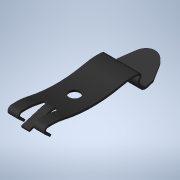
# Autodesk Inventor part: 1360395 VAME-P11-MK
Saved by Autodesk Inventor 2021 (Build 250183000, 183)
## iProperties
Created: 2026-04-23
Part Number: 1360395 VAME-P11-MK
Material: Generic
Catalog Web Link: www.3dfindit.com
Description: VAME-P11_P-h-rail mounting
Vendor: FESTO
Document SubType Name: Modeling
Designer: psAdmin
Manufacturer: FESTO
Mass: 0.583294 g
Surface Area: 16.1994 cm^2
Volume: 0.583294 cm^3
Density: 1 g/cm^3
Appearance: PSOLRGB-176-176-176
Category: PARTsolutions
Company: FESTO
Title: 1360395 VAME-P11-MK
Author: Cadenas PARTsolutions
Comments: h-rail mounting
PSOL_IDENT_0: {$CADENAS_DATA/23d-libs/festo/parts/v/vame/parts/vame_p11.prj},182 {VTYP=3D},{NB=1360395 VAME-P11-MK
PSOL_IDENT_1: },{LINA=1360395 VAME-P11-MK},{NN=VAME-P11_P},{DATE=24.07.2024 15:45:11},{GEOMDATE=16.11.2017 09:50:0
PSOL_IDENT_2: 0},{VERSION=},{LINEID=10},{WBVAR=},{WBNUMERIC=}  {NB=1360395 VAME-P11-MK},{LINA=1360395 VAME-P11-MK}
PSOL_IDENT_3: ,{KT=DUMMY},{TNR=1360395},{TYP=VAME-P11-MK}
NB: 1360395 VAME-P11-MK
NN: VAME-P11_P
NT: h-rail mounting
NBSYN: $TNR. $TYP.
LINA: 1360395 VAME-P11-MK
CATALOG: Festo
TNR: 1360395
TYP: VAME-P11-MK
SUPPLIER: FESTO
ARTICLENO: 1360395 VAME-P11-MK
BOMINFO: 1360395 VAME-P11-MK
CREATOR: CADENAS GmbH
Autodesk Inventor part; units mm, degrees
sketch "Sketch_5" plane through (0, 0, 0) normal (1, 0, 0) x (0, 1, 0)
  line L0 (10, 30) -> (-10, 30)
  line L1 (-10, 30) -> (-10, -40)
  line L2 (-10, -40) -> (10, -40)
  line L3 (10, -40) -> (10, 30)
  constraints: 8 end point
extrude "Extrusion1" add sketch "Sketch_5" along normal mid plane 14
sketch "Sketch_6" plane through (7, 0, 0) normal (1, 0, 0) x (0, 0, -1)
  line L0 (-40, 15) -> (-40, -15)
  line L1 (-40, -15) -> (50, -15)
  line L2 (50, -15) -> (50, 15)
  line L3 (50, 15) -> (-40, 15)
  arc A0 (-17.3087, 3.9004) -> (-18.3042, 1.3308) centre (-17.25, 2.4) ccw
  line L4 (-18.3042, 1.3308) -> (-16.3958, -0.3875)
  line L5 (-16.3958, -0.3875) -> (-15.8605, 0.207)
  line L6 (-15.8605, 0.207) -> (-17.7529, 1.9109)
  arc A1 (-17.3536, 3.0938) -> (-17.7529, 1.9109) centre (-17.25, 2.4) ccw
  arc A2 (-11.1052, 2.6489) -> (-17.3536, 3.0938) centre (-15.6325, -16.832) ccw
  arc A3 (-11.1052, 2.6489) -> (11.2378, 2.6792) centre (0, 51.4) ccw
  arc A4 (17.1536, 3.1033) -> (11.2378, 2.6792) centre (15.61, -16.837) ccw
  arc A5 (17.8529, 2.8657) -> (17.1536, 3.1033) centre (17.0355, 1.608) ccw
  arc A6 (17.9187, 2.2247) -> (17.8529, 2.8657) centre (17.65, 2.521) ccw
  arc A7 (17.9187, 2.2247) -> (17.3557, 0.9384) centre (18.8515, 1.05) ccw
  arc A8 (17.3557, 0.9384) -> (18.3795, -1.8266) centre (22.348, 1.215) ccw
  arc A9 (18.3795, -1.8266) -> (21.0967, -2.6739) centre (20.35, -0.288) ccw
  line L7 (21.0967, -2.6739) -> (33.0107, 1.1972)
  line L8 (33.0107, 1.1972) -> (32.7635, 1.9581)
  line L9 (32.7635, 1.9581) -> (20.8966, -1.8977)
  arc A10 (19.0122, -1.3369) -> (20.8966, -1.8977) centre (20.35, -0.288) ccw
  arc A11 (18.1515, 1.0426) -> (19.0122, -1.3369) centre (22.348, 1.215) ccw
  arc A12 (18.4278, 1.6072) -> (18.1515, 1.0426) centre (18.8515, 1.05) ccw
  arc A13 (18.4278, 1.6072) -> (18.2764, 3.5445) centre (17.65, 2.521) ccw
  arc A14 (18.2764, 3.5445) -> (17.2095, 3.9014) centre (17.0355, 1.608) ccw
  arc A15 (17.2095, 3.9014) -> (10.8828, 3.4187) centre (15.61, -16.837) ccw
  arc A16 (-11.049, 3.4567) -> (10.8828, 3.4187) centre (0, 51.4) ccw
  arc A17 (-11.049, 3.4567) -> (-17.3087, 3.9004) centre (-15.6325, -16.832) ccw
  constraints: 36 point on circle, 20 end point, 18 centre point
extrude "Extrusion2" cut sketch "Sketch_6" against normal blind 4
sketch "Sketch_7" plane through (-7, 0, 0) normal (1, 0, 0) x (0, 0, -1)
  line L0 (-40, 15) -> (-40, -15)
  line L1 (-40, -15) -> (50, -15)
  line L2 (50, -15) -> (50, 15)
  line L3 (50, 15) -> (-40, 15)
  arc A0 (-17.3087, 3.9004) -> (-18.3042, 1.3308) centre (-17.25, 2.4) ccw
  line L4 (-18.3042, 1.3308) -> (-16.3958, -0.3875)
  line L5 (-16.3958, -0.3875) -> (-15.8605, 0.207)
  line L6 (-15.8605, 0.207) -> (-17.7529, 1.9109)
  arc A1 (-17.3536, 3.0938) -> (-17.7529, 1.9109) centre (-17.25, 2.4) ccw
  arc A2 (-11.1052, 2.6489) -> (-17.3536, 3.0938) centre (-15.6325, -16.832) ccw
  arc A3 (-11.1052, 2.6489) -> (11.2378, 2.6792) centre (0, 51.4) ccw
  arc A4 (17.1536, 3.1033) -> (11.2378, 2.6792) centre (15.61, -16.837) ccw
  arc A5 (17.8529, 2.8657) -> (17.1536, 3.1033) centre (17.0355, 1.608) ccw
  arc A6 (17.9187, 2.2247) -> (17.8529, 2.8657) centre (17.65, 2.521) ccw
  arc A7 (17.9187, 2.2247) -> (17.3557, 0.9384) centre (18.8515, 1.05) ccw
  arc A8 (17.3557, 0.9384) -> (18.3795, -1.8266) centre (22.348, 1.215) ccw
  arc A9 (18.3795, -1.8266) -> (21.0967, -2.6739) centre (20.35, -0.288) ccw
  line L7 (21.0967, -2.6739) -> (33.0107, 1.1972)
  line L8 (33.0107, 1.1972) -> (32.7635, 1.9581)
  line L9 (32.7635, 1.9581) -> (20.8966, -1.8977)
  arc A10 (19.0122, -1.3369) -> (20.8966, -1.8977) centre (20.35, -0.288) ccw
  arc A11 (18.1515, 1.0426) -> (19.0122, -1.3369) centre (22.348, 1.215) ccw
  arc A12 (18.4278, 1.6072) -> (18.1515, 1.0426) centre (18.8515, 1.05) ccw
  arc A13 (18.4278, 1.6072) -> (18.2764, 3.5445) centre (17.65, 2.521) ccw
  arc A14 (18.2764, 3.5445) -> (17.2095, 3.9014) centre (17.0355, 1.608) ccw
  arc A15 (17.2095, 3.9014) -> (10.8828, 3.4187) centre (15.61, -16.837) ccw
  arc A16 (-11.049, 3.4567) -> (10.8828, 3.4187) centre (0, 51.4) ccw
  arc A17 (-11.049, 3.4567) -> (-17.3087, 3.9004) centre (-15.6325, -16.832) ccw
  constraints: 36 point on circle, 20 end point, 18 centre point
extrude "Extrusion3" cut sketch "Sketch_7" along normal blind 4
sketch "Sketch_2" plane through (0, 0, 0) normal (1, 0, 0) x (0, 1, 0)
  line L0 (-15, 40) -> (-15, -50)
  line L1 (-15, -50) -> (15, -50)
  line L2 (15, -50) -> (15, 40)
  line L3 (15, 40) -> (-15, 40)
  line L4 (0.4687, 19.036) -> (-0.2965, 18.8026)
  line L5 (-0.2965, 18.8026) -> (2.0414, 11.139)
  arc A0 (2.1693, 8.737) -> (2.0414, 11.139) centre (-2.741, 9.68) ccw
  arc A1 (2.1693, 8.737) -> (2.6792, -11.2378) centre (51.4, 0) ccw
  arc A2 (3.1033, -17.1536) -> (2.6792, -11.2378) centre (-16.837, -15.61) ccw
  arc A3 (2.8657, -17.8529) -> (3.1033, -17.1536) centre (1.608, -17.0355) ccw
  arc A4 (2.2247, -17.9187) -> (2.8657, -17.8529) centre (2.521, -17.65) ccw
  arc A5 (2.2247, -17.9187) -> (0.9384, -17.3557) centre (1.05, -18.8515) ccw
  arc A6 (0.9384, -17.3557) -> (-1.8266, -18.3795) centre (1.215, -22.348) ccw
  arc A7 (-1.8266, -18.3795) -> (-2.6739, -21.0967) centre (-0.288, -20.35) ccw
  line L6 (-2.6739, -21.0967) -> (1.1972, -33.0107)
  line L7 (1.1972, -33.0107) -> (1.9581, -32.7635)
  line L8 (1.9581, -32.7635) -> (-1.8977, -20.8966)
  arc A8 (-1.3369, -19.0122) -> (-1.8977, -20.8966) centre (-0.288, -20.35) ccw
  arc A9 (1.0426, -18.1515) -> (-1.3369, -19.0122) centre (1.215, -22.348) ccw
  arc A10 (1.6072, -18.4278) -> (1.0426, -18.1515) centre (1.05, -18.8515) ccw
  arc A11 (1.6072, -18.4278) -> (3.5445, -18.2764) centre (2.521, -17.65) ccw
  arc A12 (3.5445, -18.2764) -> (3.9014, -17.2095) centre (1.608, -17.0355) ccw
  arc A13 (3.9014, -17.2095) -> (3.4187, -10.8828) centre (-16.837, -15.61) ccw
  arc A14 (2.9801, 8.7267) -> (3.4187, -10.8828) centre (51.4, 0) ccw
  arc A15 (2.9801, 8.7267) -> (2.8066, 11.3724) centre (-2.741, 9.68) ccw
  line L9 (2.8066, 11.3724) -> (0.4687, 19.036)
  constraints: 32 point on circle, 20 end point, 16 centre point
extrude "Extrusion4" cut sketch "Sketch_2" along normal mid plane 6
sketch "Sketch_3" plane through (0, 0, 0) normal (0, 1, 0) x (-1, 0, 0)
  line L0 (3, 28.8) -> (-3, 28.8)
  line L1 (-3, 28.8) -> (-3, 8.8)
  line L2 (-3, 8.8) -> (-1.5, 8.8)
  line L3 (-1.5, 8.8) -> (-1.5, 26.8)
  line L4 (-1.5, 26.8) -> (1.5, 26.8)
  line L5 (1.5, 26.8) -> (1.5, 8.8)
  line L6 (1.5, 8.8) -> (3, 8.8)
  line L7 (3, 8.8) -> (3, 28.8)
  constraints: 16 end point
extrude "Extrusion5" cut sketch "Sketch_3" along normal mid plane 16
sketch "Sketch_1" plane through (0, 0, 0) normal (0, 1, 0) x (-1, 0, 0)
  line L0 (7, -35.341) -> (7, -23.341)
  line L1 (7, -23.341) -> (4.55, -28.1703)
  arc A0 (-4.55, -28.1703) -> (4.55, -28.1703) centre (0, -25.862) ccw
  line L2 (-4.55, -28.1703) -> (-7, -23.341)
  line L3 (-7, -23.341) -> (-7, -35.341)
  line L4 (-7, -35.341) -> (7, -35.341)
  constraints: 10 end point, 2 point on circle, 1 centre point
extrude "Extrusion6" cut sketch "Sketch_1" along normal mid plane 16
sketch "Sketch_8" plane through (0, 0, 0) normal (0, 0, 1) x (1, 0, 0)
  line L0 (0, 1.4) -> (0, 2.5)
  line L1 (0, 2.5) -> (2.1, 2.5)
  line L2 (2.1, 2.5) -> (2.1, 1.4)
  line L3 (2.1, 1.4) -> (0, 1.4)
  line L4 (0, 1.4) -> (0, 2.5)
  constraints: 10 end point
revolve "Revolution1" cut sketch "Sketch_8" angle 360 about axis through (0, 1.4, 0) along (0, -1, 0)
ref_plane "ANBAU_XY" through (0, 0, 0) normal (-1, 0, 0) x (0, 0, -1)
ref_plane "ANBAU_YZ" through (0, 0, 0) normal (0, 0, -1) x (0, -1, 0)
ref_plane "ANBAU_ZX" through (0, 0, 0) normal (0, -1, 0) x (-1, 0, 0)
ref_plane "B_XY" through (0, 1.4, 0) normal (0, -1, 0) x (1, 0, 0)
ref_plane "B_YZ" through (0, 1.4, 0) normal (1, 0, 0) x (0, 0, 1)
ref_plane "B_ZX" through (0, 1.4, 0) normal (0, 0, 1) x (0, -1, 0)
ref_plane "N_XY" through (0, 2.6, 0) normal (0, 1, 0) x (1, 0, 0)
ref_plane "N_YZ" through (0, 2.6, 0) normal (1, 0, 0) x (0, 0, -1)
ref_plane "N_ZX" through (0, 2.6, 0) normal (0, 0, -1) x (0, 1, 0)
body "Solid1"
